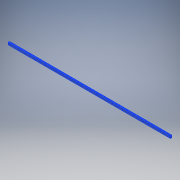
# Autodesk Inventor part: SRS12M7907.5 Track
Saved by Autodesk Inventor 2016 (Build 200138000, 138)
## iProperties
Category: PARTsolutions
Company: THK
Created: 2015-05-12
Part Number: SRS12M7907.5 Track
Catalog Web Link: www.cadenas.de
Description: Compact Type SRS-M Track-SHW-CA
Vendor: THK
Document SubType Name: Modeling
Designer: PARTuser1
Manufacturer: THK
Mass: 508.696 g
Surface Area: 342.81 cm^2
Volume: 63.587 cm^3
Density: 8 g/cm^3
Material: Stainless Steel
Appearance: Semi-Polished
PSOL_IDENT_0: {$CADENAS_DATA\23d-libs\thk\linear_motion_systems\lm_guide\lm_caged_ball_roller\caged_ball\lm_guide_
PSOL_IDENT_1: srs\srs_m\srs_m_track.prj},203 {VTYP=3D},{NB=SRS12M7907.5 Track},{LINA=SRS12M7907.5 Track},{NN=Compa
PSOL_IDENT_2: ct Type SRS-M Track},{DATE=12.05.2014 11:34:27},{GEOMDATE=12.05.2014 11:34:27},{VERSION=},{LINEID=12
PSOL_IDENT_3: 0},{LINESUBID=-1},{WBVAR=L,G,GX}  {NB=SRS12M7907.5 Track},{LINA=SRS12M7907.5 Track},{KT=DUMMY},{MN=S
PSOL_IDENT_4: RS12M},{ND=3.000},{NOB=1},{L=790.0},{G=},{GG='', 'Symmetrical (G1=G2)', 'A', 'Asymmetrical'},{GX=7.5
PSOL_IDENT_5: },{GX1=7.5},{LMIN=34.4},{LEND=3885.00},{LMING=4.00},{LMAXG=16.00},{M=13.00},{W=27.00},{LTR=34.40},{H
PSOL_IDENT_6: 3=2.00},{W1=12.00},{W2=7.50},{M1=7.50},{F=25.00},{D1=3.50},{D2=6.00},{HM=4.50},{MAXL=1340.00},{GMIN=
PSOL_IDENT_7: 4},{GMX=7.5},{GMAX1=31.28},{G1=7.5},{G2=7.5},{NX=1},{A=32},{LF=-5},{LM=800},{LL=1595},{AA=31},{GMAX=
PSOL_IDENT_8: 11},{P=32},{PX=0},{VG=31},{VGG=7.5},{VG1=-1},{VG2=32},{LT=1295},{GA=10.000}
SUPPLIER: THK
ARTICLENO: SRS12M7907.5 Track
BOMINFO: SRS12M7907.5 Track
CREATOR: CADENAS GmbH
Title: SRS12M7907.5 Track
Author: Cadenas PARTsolutions
Comments: SHW-CA
Autodesk Inventor part; units mm, degrees
ref_plane "YZ Plane" through (0, 0, 0) normal (1, 0, 0) x (0, 1, 0)
ref_plane "XZ Plane" through (0, 0, 0) normal (0, 1, 0) x (-1, 0, 0)
ref_plane "XY Plane" through (0, 0, 0) normal (0, 0, 1) x (1, 0, 0)
sketch "Sketch_3" plane through (-7.5, 0, 0) normal (1, 0, 0) x (0, 0, -1)
  line L0 (-6, 0.5) -> (-5.5, 0)
  line L1 (-5.5, 0) -> (5.5, 0)
  line L2 (5.5, 0) -> (6, 0.5)
  line L3 (6, 0.5) -> (6, 3.9874)
  arc A0 (5.2629, 5.3) -> (6, 3.9874) centre (6.64, 5.21) ccw
  arc A1 (6, 6.6126) -> (5.2629, 5.3) centre (6.64, 5.39) ccw
  line L4 (6, 6.6126) -> (6, 7.2)
  line L5 (6, 7.2) -> (5.7, 7.5)
  line L6 (5.7, 7.5) -> (-5.7, 7.5)
  line L7 (-5.7, 7.5) -> (-6, 7.2)
  line L8 (-6, 7.2) -> (-6, 6.6126)
  arc A2 (-5.2629, 5.3) -> (-6, 6.6126) centre (-6.64, 5.39) ccw
  arc A3 (-6, 3.9874) -> (-5.2629, 5.3) centre (-6.64, 5.21) ccw
  line L9 (-6, 3.9874) -> (-6, 0.5)
  constraints: 20 end point, 8 point on circle, 4 centre point
extrude "Extrusion1" add sketch "Sketch_3" along normal blind 790
sketch "Sketch2" plane through (-7.5, 7.5, -5.7) normal (0, 1, 0) x (1, 0, 0)
  point P0 (7.5, -5.7)
hole "Hole1" at (0, 7.5, 0) direction (0, -1, 0) diameter 3.5 depth 7.5 counterbore diameter 6 counterbore depth 4.5
pattern_linear "Rectangular Pattern1" count 32 spacing 25 along (1, 0, 0) of "Hole1"
ref_plane "4dummy_XY" through (0, 0, 0) normal (1, 0, 0) x (0, 0, -1)
ref_plane "4dummy_YZ" through (0, 0, 0) normal (0, 0, -1) x (0, 1, 0)
ref_plane "4dummy_ZX" through (0, 0, 0) normal (0, 1, 0) x (1, 0, 0)
ref_plane "4slide_XY" through (-7.5, 2, 0) normal (1, 0, 0) x (0, 0, -1)
ref_plane "4slide_YZ" through (-7.5, 2, 0) normal (0, 0, -1) x (0, 1, 0)
ref_plane "4slide_ZX" through (-7.5, 2, 0) normal (0, 1, 0) x (1, 0, 0)
ref_plane "4track_XY" through (0, 0, 0) normal (0, 0, 1) x (1, 0, 0)
ref_plane "4track_YZ" through (0, 0, 0) normal (1, 0, 0) x (0, 1, 0)
ref_plane "4track_ZX" through (0, 0, 0) normal (0, 1, 0) x (0, 0, 1)
body "Solid1"
